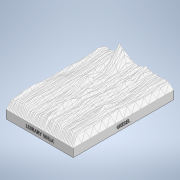
# Autodesk Inventor part: 12_tone_fourier_transform
Saved by Autodesk Inventor 2020 (Build 240168000, 168)
## iProperties
Created: 2019-10-01
Part Number: 12_tone_fourier_transform
Material: Generic
Document SubType Name: Modeling
Designer: Babynado
Density: 1 g/cm^3
Appearance: Default
Author: Babynado
Autodesk Inventor part; units mm, degrees
(part 1 of 4)
ref_plane "YZ Plane" through (0, 0, 0) normal (1, 0, 0) x (0, 1, 0)
ref_plane "XZ Plane" through (0, 0, 0) normal (0, 1, 0) x (-1, 0, 0)
ref_plane "XY Plane" through (0, 0, 0) normal (0, 0, 1) x (1, 0, 0)
sketch "Sketch1" plane through (0, 0, 0) normal (0, 1, 0) x (-1, 0, 0)
  line L0 (-203.2, 304.8) -> (-203.2, 0) projected
  line L1 (0, 304.8) -> (-203.2, 304.8) projected
  line L2 (0, 0) -> (0, 304.8) projected
  line L3 (-203.2, 0) -> (0, 0) projected
extrude "Extrusion1" add sketch "Sketch1" against normal blind 25.4
sketch "Sketch2" plane through (0, 0, 304.8) normal (0, 0, 1) x (1, 0, 0)
  line L0 (0, 0) -> (203.2, 0) projected
  line L1 (0, 0) -> (0, -25.4) projected
  line L2 (203.2, -25.4) -> (0, -25.4) projected
  line L3 (203.2, 0) -> (203.2, -25.4) projected
  line L4 (50.8, -8.636) -> (152.4, -8.636) construction
  line L5 (152.4, -8.636) -> (152.4, -16.764) construction
  line L6 (152.4, -16.764) -> (50.8, -16.764) construction
  line L7 (50.8, -16.764) -> (50.8, -8.636) construction
  line L8 (65.2204, -17.272) -> (59.9222, -17.272)
  line L9 (59.9222, -17.272) -> (59.9222, -8.128)
  line L10 (59.9222, -8.128) -> (61.1374, -8.128)
  line L11 (61.1374, -8.128) -> (61.1374, -16.1901)
  line L12 (61.1374, -16.1901) -> (65.2204, -16.1901)
  line L13 (65.2204, -16.1901) -> (65.2204, -17.272)
  line L14 (69.3626, -17.272) -> (65.8206, -17.272)
  line L15 (65.8206, -17.272) -> (65.8206, -16.3383)
  line L16 (65.8206, -16.3383) -> (66.984, -16.3383)
  line L17 (66.984, -16.3383) -> (66.984, -9.0617)
  line L18 (66.984, -9.0617) -> (65.8206, -9.0617)
  line L19 (65.8206, -9.0617) -> (65.8206, -8.128)
  line L20 (65.8206, -8.128) -> (69.3626, -8.128)
  line L21 (69.3626, -8.128) -> (69.3626, -9.0617)
  line L22 (69.3626, -9.0617) -> (68.1992, -9.0617)
  line L23 (68.1992, -9.0617) -> (68.1992, -16.3383)
  line L24 (68.1992, -16.3383) -> (69.3626, -16.3383)
  line L25 (69.3626, -16.3383) -> (69.3626, -17.272)
  spline S0 degree 2 poles (77.069, -14.4636) (77.069, -15.1453) (76.5503, -16.1901) (76.1205, -16.531) knots 0 0 0 1 2 2 2
  spline S1 degree 2 poles (76.1205, -16.531) (75.6018, -16.9311) (74.4236, -17.272) (73.49, -17.272) knots 0 0 0 1 2 2 2
  line L26 (73.49, -17.272) -> (70.8668, -17.272)
  line L27 (70.8668, -17.272) -> (70.8668, -8.128)
  line L28 (70.8668, -8.128) -> (73.2899, -8.128)
  spline S2 degree 2 poles (73.2899, -8.128) (74.268, -8.128) (75.2462, -8.254) (75.6908, -8.4985) knots 0 0 0 1 2 2 2
  spline S3 degree 2 poles (75.6908, -8.4985) (76.1872, -8.7579) (76.6392, -9.61) (76.6392, -10.188) knots 0 0 0 1 2 2 2
  spline S4 degree 2 poles (76.6392, -10.188) (76.6392, -10.8327) (75.9575, -11.8553) (75.3573, -12.1442) knots 0 0 0 1 2 2 2
  line L29 (75.3573, -12.1442) -> (75.3573, -12.1887)
  spline S5 degree 2 poles (75.3573, -12.1887) (76.1724, -12.411) (77.069, -13.5892) (77.069, -14.4636) knots 0 0 0 1 2 2 2
  spline S6 degree 2 poles (75.8019, -14.5155) (75.8019, -13.9968) (75.5055, -13.3299) (75.0609, -13.0927) knots 0 0 0 1 2 2 2
  spline S7 degree 2 poles (75.0609, -13.0927) (74.7719, -12.9445) (74.0902, -12.8556) (73.4603, -12.8556) knots 0 0 0 1 2 2 2
  line L30 (73.4603, -12.8556) -> (72.0821, -12.8556)
  line L31 (72.0821, -12.8556) -> (72.0821, -16.2346)
  line L32 (72.0821, -16.2346) -> (73.0676, -16.2346)
  spline S8 degree 2 poles (73.0676, -16.2346) (73.8679, -16.2346) (74.7867, -16.0864) (75.1424, -15.8493) knots 0 0 0 1 2 2 2
  spline S9 degree 2 poles (75.1424, -15.8493) (75.4833, -15.6047) (75.8019, -14.9971) (75.8019, -14.5155) knots 0 0 0 1 2 2 2
  spline S10 degree 2 poles (75.3721, -10.3584) (75.3721, -10.0324) (75.1498, -9.5433) (74.9053, -9.4025) knots 0 0 0 1 2 2 2
  spline S11 degree 2 poles (74.9053, -9.4025) (74.6089, -9.2395) (73.8901, -9.1654) (73.2454, -9.1654) knots 0 0 0 1 2 2 2
  line L33 (73.2454, -9.1654) -> (72.0821, -9.1654)
  line L34 (72.0821, -9.1654) -> (72.0821, -11.8404)
  line L35 (72.0821, -11.8404) -> (73.4603, -11.8404)
  spline S12 degree 2 poles (73.4603, -11.8404) (74.0309, -11.8404) (74.5718, -11.7219) (74.8608, -11.5366) knots 0 0 0 1 2 2 2
  spline S13 degree 2 poles (74.8608, -11.5366) (75.1424, -11.3588) (75.3721, -10.7882) (75.3721, -10.3584) knots 0 0 0 1 2 2 2
  line L36 (85.3535, -17.272) -> (83.7751, -17.272)
  line L37 (83.7751, -17.272) -> (80.8852, -13.6337)
  line L38 (80.8852, -13.6337) -> (79.4921, -13.6337)
  line L39 (79.4921, -13.6337) -> (79.4921, -17.272)
  line L40 (79.4921, -17.272) -> (78.2769, -17.272)
  line L41 (78.2769, -17.272) -> (78.2769, -8.128)
  line L42 (78.2769, -8.128) -> (80.6333, -8.128)
  spline S14 degree 2 poles (80.6333, -8.128) (81.4187, -8.128) (82.4784, -8.2984) (82.96, -8.6097) knots 0 0 0 1 2 2 2
  spline S15 degree 2 poles (82.96, -8.6097) (83.4417, -8.9209) (83.9974, -9.8916) (83.9974, -10.6104) knots 0 0 0 1 2 2 2
  spline S16 degree 2 poles (83.9974, -10.6104) (83.9974, -11.6107) (82.9748, -12.9668) (82.1005, -13.2928) knots 0 0 0 1 2 2 2
  line L43 (82.1005, -13.2928) -> (85.3535, -17.272)
  spline S17 degree 2 poles (82.7303, -10.7067) (82.7303, -10.3066) (82.4487, -9.6915) (82.1523, -9.4914) knots 0 0 0 1 2 2 2
  spline S18 degree 2 poles (82.1523, -9.4914) (81.893, -9.321) (81.2038, -9.1802) (80.7, -9.1802) knots 0 0 0 1 2 2 2
  line L44 (80.7, -9.1802) -> (79.4921, -9.1802)
  line L45 (79.4921, -9.1802) -> (79.4921, -12.6185)
  line L46 (79.4921, -12.6185) -> (80.5592, -12.6185)
  spline S19 degree 2 poles (80.5592, -12.6185) (81.0853, -12.6185) (81.9226, -12.4332) (82.2116, -12.1442) knots 0 0 0 1 2 2 2
  spline S20 degree 2 poles (82.2116, -12.1442) (82.4784, -11.8923) (82.7303, -11.1809) (82.7303, -10.7067) knots 0 0 0 1 2 2 2
  line L47 (85.0941, -17.272) -> (88.1767, -8.128)
  line L48 (88.1767, -8.128) -> (89.6735, -8.128)
  line L49 (89.6735, -8.128) -> (92.7561, -17.272)
  line L50 (92.7561, -17.272) -> (91.4742, -17.272)
  line L51 (91.4742, -17.272) -> (90.6442, -14.7155)
  line L52 (90.6442, -14.7155) -> (87.1541, -14.7155)
  line L53 (87.1541, -14.7155) -> (86.3242, -17.272)
  line L54 (86.3242, -17.272) -> (85.0941, -17.272)
  line L55 (90.3108, -13.6781) -> (88.8955, -9.3729)
  line L56 (88.8955, -9.3729) -> (87.4876, -13.6781)
  line L57 (87.4876, -13.6781) -> (90.3108, -13.6781)
  line L58 (100.6997, -17.272) -> (99.1213, -17.272)
  line L59 (99.1213, -17.272) -> (96.2314, -13.6337)
  line L60 (96.2314, -13.6337) -> (94.8383, -13.6337)
  line L61 (94.8383, -13.6337) -> (94.8383, -17.272)
  line L62 (94.8383, -17.272) -> (93.6231, -17.272)
  line L63 (93.6231, -17.272) -> (93.6231, -8.128)
  line L64 (93.6231, -8.128) -> (95.9795, -8.128)
  spline S21 degree 2 poles (95.9795, -8.128) (96.7649, -8.128) (97.8246, -8.2984) (98.3062, -8.6097) knots 0 0 0 1 2 2 2
  spline S22 degree 2 poles (98.3062, -8.6097) (98.7879, -8.9209) (99.3436, -9.8916) (99.3436, -10.6104) knots 0 0 0 1 2 2 2
  spline S23 degree 2 poles (99.3436, -10.6104) (99.3436, -11.6107) (98.3211, -12.9668) (97.4467, -13.2928) knots 0 0 0 1 2 2 2
  line L65 (97.4467, -13.2928) -> (100.6997, -17.272)
  spline S24 degree 2 poles (98.0765, -10.7067) (98.0765, -10.3066) (97.7949, -9.6915) (97.4985, -9.4914) knots 0 0 0 1 2 2 2
  spline S25 degree 2 poles (97.4985, -9.4914) (97.2392, -9.321) (96.55, -9.1802) (96.0462, -9.1802) knots 0 0 0 1 2 2 2
  line L66 (96.0462, -9.1802) -> (94.8383, -9.1802)
  line L67 (94.8383, -9.1802) -> (94.8383, -12.6185)
  line L68 (94.8383, -12.6185) -> (95.9054, -12.6185)
  spline S26 degree 2 poles (95.9054, -12.6185) (96.4315, -12.6185) (97.2688, -12.4332) (97.5578, -12.1442) knots 0 0 0 1 2 2 2
  spline S27 degree 2 poles (97.5578, -12.1442) (97.8246, -11.8923) (98.0765, -11.1809) (98.0765, -10.7067) knots 0 0 0 1 2 2 2
  line L69 (107.8281, -8.128) -> (104.7382, -13.2261)
  line L70 (104.7382, -13.2261) -> (104.7382, -17.272)
  line L71 (104.7382, -17.272) -> (103.5229, -17.272)
  line L72 (103.5229, -17.272) -> (103.5229, -13.3521)
  line L73 (103.5229, -13.3521) -> (100.4329, -8.128)
  line L74 (100.4329, -8.128) -> (101.7815, -8.128)
  line L75 (101.7815, -8.128) -> (104.1379, -12.1517)
  line L76 (104.1379, -12.1517) -> (106.5388, -8.128)
  line L77 (106.5388, -8.128) -> (107.8281, -8.128)
  line L78 (122.8483, -8.128) -> (120.5512, -17.272)
  line L79 (120.5512, -17.272) -> (119.1877, -17.272)
  line L80 (119.1877, -17.272) -> (117.3278, -9.6841)
  line L81 (117.3278, -9.6841) -> (115.5198, -17.272)
  line L82 (115.5198, -17.272) -> (114.1711, -17.272)
  line L83 (114.1711, -17.272) -> (111.837, -8.128)
  line L84 (111.837, -8.128) -> (113.0893, -8.128)
  line L85 (113.0893, -8.128) -> (114.927, -15.7085)
  line L86 (114.927, -15.7085) -> (116.7498, -8.128)
  line L87 (116.7498, -8.128) -> (117.9873, -8.128)
  line L88 (117.9873, -8.128) -> (119.825, -15.7974)
  line L89 (119.825, -15.7974) -> (121.6553, -8.128)
  line L90 (121.6553, -8.128) -> (122.8483, -8.128)
  line L91 (122.9521, -17.272) -> (126.0346, -8.128)
  line L92 (126.0346, -8.128) -> (127.5315, -8.128)
  line L93 (127.5315, -8.128) -> (130.614, -17.272)
  line L94 (130.614, -17.272) -> (129.3321, -17.272)
  line L95 (129.3321, -17.272) -> (128.5022, -14.7155)
  line L96 (128.5022, -14.7155) -> (125.012, -14.7155)
  line L97 (125.012, -14.7155) -> (124.1821, -17.272)
  line L98 (124.1821, -17.272) -> (122.9521, -17.272)
  line L99 (128.1687, -13.6781) -> (126.7534, -9.3729)
  line L100 (126.7534, -9.3729) -> (125.3455, -13.6781)
  line L101 (125.3455, -13.6781) -> (128.1687, -13.6781)
  line L102 (136.7792, -17.272) -> (131.481, -17.272)
  line L103 (131.481, -17.272) -> (131.481, -8.128)
  line L104 (131.481, -8.128) -> (132.6963, -8.128)
  line L105 (132.6963, -8.128) -> (132.6963, -16.1901)
  line L106 (132.6963, -16.1901) -> (136.7792, -16.1901)
  line L107 (136.7792, -16.1901) -> (136.7792, -17.272)
  line L108 (144.4041, -17.272) -> (142.8258, -17.272)
  line L109 (142.8258, -17.272) -> (139.4839, -13.0186)
  line L110 (139.4839, -13.0186) -> (138.9503, -13.6188)
  line L111 (138.9503, -13.6188) -> (138.9503, -17.272)
  line L112 (138.9503, -17.272) -> (137.7351, -17.272)
  line L113 (137.7351, -17.272) -> (137.7351, -8.128)
  line L114 (137.7351, -8.128) -> (138.9503, -8.128)
  line L115 (138.9503, -8.128) -> (138.9503, -12.3295)
  line L116 (138.9503, -12.3295) -> (142.6998, -8.128)
  line L117 (142.6998, -8.128) -> (144.1818, -8.128)
  line L118 (144.1818, -8.128) -> (140.3953, -12.2109)
  line L119 (140.3953, -12.2109) -> (144.4041, -17.272)
  dimension "d2" = 203.2
  dimension "d3" = 25.4
  dimension "d4" = 101.6
  dimension "d5" = 8.128
  dimension "d6" = 50.8
  dimension "d7" = 8.636
  constraints: 2 other
  measures "d2" distance of L0.start L0.end
  measures "d3" distance of L0.start L1.end
  measures "d4" distance of L4.start L4.end
  measures "d5" distance of L6.end L4.start
  measures "d6" distance between parallel lines of L1 L7
  measures "d7" distance between parallel lines of L2 L6
extrude "Extrusion2" cut sketch "Sketch2" against normal blind 5.08 contours L8 L9 L10 L11 L12 L13 | L14 L15 L16 L17 L18 L19 L20 L21 L22 L23 L24 L25 | S0 S1 L26 L27 L28 S2 S3 S4 L29 S5 | L36 L47 L43 | L43 L47 L48 L49 L50 L51 L52 L53 L54 | L36 L37 L38 L39 L40 L41 L42 S14 S15 S16 L43 L47 | L58 L59 L60 L61 L62 L63 L64 S21 S22 S23 L65 | L69 L70 L71 L72 L73 L74 L75 L76 L77 | L78 L79 L80 L81 L82 L83 L84 L85 L86 L87 L88 L89 L90 | L91 L92 L93 L94 L95 L96 L97 L98 | L102 L103 L104 L105 L106 L107 | L108 L109 L110 L111 L112 L113 L114 L115 L116 L117 L118 L119
sketch "Sketch3" plane through (203.2, 0, 304.8) normal (1, 0, 0) x (0, 0, -1)
  line L0 (0, 0) -> (304.8, 0) projected
  line L1 (0, 0) -> (0, -25.4) projected
  line L2 (304.8, -25.4) -> (0, -25.4) projected
  line L3 (304.8, 0) -> (304.8, -25.4) projected
  line L4 (120.65, -8.636) -> (184.15, -8.636) construction
  line L5 (184.15, -8.636) -> (184.15, -16.764) construction
  line L6 (184.15, -16.764) -> (120.65, -16.764) construction
  line L7 (120.65, -16.764) -> (120.65, -8.636) construction
  spline S0 degree 2 poles (136.9315, -17.4424) (135.9608, -17.4424) (134.3528, -16.8496) (133.7748, -16.2494) knots 0 0 0 1 2 2 2
  spline S1 degree 2 poles (133.7748, -16.2494) (133.1969, -15.6418) (132.5818, -13.8486) (132.5818, -12.6852) knots 0 0 0 1 2 2 2
  spline S2 degree 2 poles (132.5818, -12.6852) (132.5818, -11.5811) (133.2043, -9.8323) (133.7823, -9.2099) knots 0 0 0 1 2 2 2
  spline S3 degree 2 poles (133.7823, -9.2099) (134.338, -8.6097) (135.9682, -7.9576) (136.9389, -7.9576) knots 0 0 0 1 2 2 2
  spline S4 degree 2 poles (136.9389, -7.9576) (137.4058, -7.9576) (138.2505, -8.0909) (138.6358, -8.2095) knots 0 0 0 1 2 2 2
  spline S5 degree 2 poles (138.6358, -8.2095) (138.9471, -8.2984) (139.7029, -8.6245) (139.9326, -8.743) knots 0 0 0 1 2 2 2
  line L8 (139.9326, -8.743) -> (139.9326, -10.2102)
  line L9 (139.9326, -10.2102) -> (139.8289, -10.2102)
  spline S6 degree 2 poles (139.8289, -10.2102) (139.5991, -10.0102) (139.1175, -9.6471) (138.6729, -9.4396) knots 0 0 0 1 2 2 2
  spline S7 degree 2 poles (138.6729, -9.4396) (138.3024, -9.2543) (137.3465, -9.0098) (136.7981, -9.0098) knots 0 0 0 1 2 2 2
  spline S8 degree 2 poles (136.7981, -9.0098) (135.4792, -9.0098) (133.8489, -10.9957) (133.8489, -12.6481) knots 0 0 0 1 2 2 2
  spline S9 degree 2 poles (133.8489, -12.6481) (133.8489, -13.567) (134.2787, -14.9452) (134.6863, -15.4195) knots 0 0 0 1 2 2 2
  spline S10 degree 2 poles (134.6863, -15.4195) (135.079, -15.8937) (136.1905, -16.3902) (136.8871, -16.3902) knots 0 0 0 1 2 2 2
  spline S11 degree 2 poles (136.8871, -16.3902) (137.3984, -16.3902) (138.4209, -16.242) (138.7692, -16.0938) knots 0 0 0 1 2 2 2
  line L10 (138.7692, -16.0938) -> (138.7692, -13.73)
  line L11 (138.7692, -13.73) -> (136.6499, -13.73)
  line L12 (136.6499, -13.73) -> (136.6499, -12.6629)
  line L13 (136.6499, -12.6629) -> (139.9696, -12.6629)
  line L14 (139.9696, -12.6629) -> (139.9696, -16.657)
  spline S12 degree 2 poles (139.9696, -16.657) (139.7399, -16.7607) (138.9545, -17.0793) (138.621, -17.1757) knots 0 0 0 1 2 2 2
  spline S13 degree 2 poles (138.621, -17.1757) (138.169, -17.3091) (137.4428, -17.4424) (136.9315, -17.4424) knots 0 0 0 1 2 2 2
  line L15 (141.4961, -17.2646) -> (141.4961, -8.1206)
  line L16 (141.4961, -8.1206) -> (147.2167, -8.1206)
  line L17 (147.2167, -8.1206) -> (147.2167, -9.2025)
  line L18 (147.2167, -9.2025) -> (142.7114, -9.2025)
  line L19 (142.7114, -9.2025) -> (142.7114, -11.7071)
  line L20 (142.7114, -11.7071) -> (146.9129, -11.7071)
  line L21 (146.9129, -11.7071) -> (146.9129, -12.7889)
  line L22 (146.9129, -12.7889) -> (142.7114, -12.7889)
  line L23 (142.7114, -12.7889) -> (142.7114, -16.1827)
  line L24 (142.7114, -16.1827) -> (147.2167, -16.1827)
  line L25 (147.2167, -16.1827) -> (147.2167, -17.2646)
  line L26 (147.2167, -17.2646) -> (141.4961, -17.2646)
  line L27 (151.7368, -17.2646) -> (148.1948, -17.2646)
  line L28 (148.1948, -17.2646) -> (148.1948, -16.3309)
  line L29 (148.1948, -16.3309) -> (149.3582, -16.3309)
  line L30 (149.3582, -16.3309) -> (149.3582, -9.0543)
  line L31 (149.3582, -9.0543) -> (148.1948, -9.0543)
  line L32 (148.1948, -9.0543) -> (148.1948, -8.1206)
  line L33 (148.1948, -8.1206) -> (151.7368, -8.1206)
  line L34 (151.7368, -8.1206) -> (151.7368, -9.0543)
  line L35 (151.7368, -9.0543) -> (150.5734, -9.0543)
  line L36 (150.5734, -9.0543) -> (150.5734, -16.3309)
  line L37 (150.5734, -16.3309) -> (151.7368, -16.3309)
  line L38 (151.7368, -16.3309) -> (151.7368, -17.2646)
  spline S14 degree 2 poles (155.7901, -17.4276) (154.7971, -17.4276) (153.4041, -17.0126) (152.789, -16.7162) knots 0 0 0 1 2 2 2
  line L39 (152.789, -16.7162) -> (152.789, -15.1898)
  line L40 (152.789, -15.1898) -> (152.8779, -15.1898)
  spline S15 degree 2 poles (152.8779, -15.1898) (153.4782, -15.7529) (154.9972, -16.3754) (155.7012, -16.3754) knots 0 0 0 1 2 2 2
  spline S16 degree 2 poles (155.7012, -16.3754) (156.7089, -16.3754) (157.7389, -15.538) (157.7389, -14.8489) knots 0 0 0 1 2 2 2
  spline S17 degree 2 poles (157.7389, -14.8489) (157.7389, -14.3006) (157.198, -13.6188) (156.6126, -13.4484) knots 0 0 0 1 2 2 2
  spline S18 degree 2 poles (156.6126, -13.4484) (156.1902, -13.3299) (155.4863, -13.1668) (154.9602, -13.0335) knots 0 0 0 1 2 2 2
  spline S19 degree 2 poles (154.9602, -13.0335) (154.4859, -12.9075) (153.7375, -12.5296) (153.4485, -12.2258) knots 0 0 0 1 2 2 2
  spline S20 degree 2 poles (153.4485, -12.2258) (153.1669, -11.9219) (152.8557, -11.1068) (152.8557, -10.5733) knots 0 0 0 1 2 2 2
  spline S21 degree 2 poles (152.8557, -10.5733) (152.8557, -9.4618) (154.5897, -7.9576) (155.9309, -7.9576) knots 0 0 0 1 2 2 2
  spline S22 degree 2 poles (155.9309, -7.9576) (156.7015, -7.9576) (158.065, -8.2614) (158.6504, -8.5504) knots 0 0 0 1 2 2 2
  line L41 (158.6504, -8.5504) -> (158.6504, -10.0027)
  line L42 (158.6504, -10.0027) -> (158.5615, -10.0027)
  spline S23 degree 2 poles (158.5615, -10.0027) (158.1243, -9.6026) (156.7608, -9.0098) (156.0124, -9.0098) knots 0 0 0 1 2 2 2
  spline S24 degree 2 poles (156.0124, -9.0098) (155.1677, -9.0098) (154.1228, -9.8027) (154.1228, -10.4473) knots 0 0 0 1 2 2 2
  spline S25 degree 2 poles (154.1228, -10.4473) (154.1228, -11.0253) (154.7379, -11.7145) (155.3159, -11.8701) knots 0 0 0 1 2 2 2
  spline S26 degree 2 poles (155.3159, -11.8701) (155.7012, -11.9738) (156.8201, -12.2406) (157.1906, -12.3517) knots 0 0 0 1 2 2 2
  spline S27 degree 2 poles (157.1906, -12.3517) (158.1317, -12.6407) (159.0061, -13.8041) (159.0061, -14.6563) knots 0 0 0 1 2 2 2
  spline S28 degree 2 poles (159.0061, -14.6563) (159.0061, -15.1972) (158.5689, -16.2346) (158.1761, -16.5977) knots 0 0 0 1 2 2 2
  spline S29 degree 2 poles (158.1761, -16.5977) (157.7389, -16.9978) (156.6274, -17.4276) (155.7901, -17.4276) knots 0 0 0 1 2 2 2
  line L43 (160.2435, -17.2646) -> (160.2435, -8.1206)
  line L44 (160.2435, -8.1206) -> (165.9641, -8.1206)
  line L45 (165.9641, -8.1206) -> (165.9641, -9.2025)
  line L46 (165.9641, -9.2025) -> (161.4588, -9.2025)
  line L47 (161.4588, -9.2025) -> (161.4588, -11.7071)
  line L48 (161.4588, -11.7071) -> (165.6603, -11.7071)
  line L49 (165.6603, -11.7071) -> (165.6603, -12.7889)
  line L50 (165.6603, -12.7889) -> (161.4588, -12.7889)
  line L51 (161.4588, -12.7889) -> (161.4588, -16.1827)
  line L52 (161.4588, -16.1827) -> (165.9641, -16.1827)
  line L53 (165.9641, -16.1827) -> (165.9641, -17.2646)
  line L54 (165.9641, -17.2646) -> (160.2435, -17.2646)
  line L55 (172.5961, -17.2646) -> (167.2979, -17.2646)
  line L56 (167.2979, -17.2646) -> (167.2979, -8.1206)
  line L57 (167.2979, -8.1206) -> (168.5131, -8.1206)
  line L58 (168.5131, -8.1206) -> (168.5131, -16.1827)
  line L59 (168.5131, -16.1827) -> (172.5961, -16.1827)
  line L60 (172.5961, -16.1827) -> (172.5961, -17.2646)
  dimension "d10" = 304.8
  dimension "d11" = 25.4
  dimension "d12" = 63.5
  dimension "d13" = 8.128
  dimension "d14" = 120.65
  dimension "d15" = 8.636
  constraints: 2 other
  measures "d10" distance of L0.start L0.end
  measures "d11" distance of L0.start L1.end
  measures "d12" distance of L4.start L4.end
  measures "d13" distance of L6.end L4.start
  measures "d14" distance between parallel lines of L1 L7
  measures "d15" distance between parallel lines of L2 L6
extrude "Extrusion3" cut sketch "Sketch3" against normal blind 5.08 contours S0 S1 S2 S3 S4 S5 L8 L9 S6 S7 S8 S9 S10 S11 L10 L11 L12 L13 L14 S12 S13 | L15 L16 L17 L18 L19 L20 L21 L22 L23 L24 L25 L26 | L27 L28 L29 L30 L31 L32 L33 L34 L35 L36 L37 L38 | S14 L39 L40 S15 S16 S17 S18 S19 S20 S21 S22 L41 L42 S23 S24 S25 S26 S27 S28 S29 | L43 L44 L45 L46 L47 L48 L49 L50 L51 L52 L53 L54 | L55 L56 L57 L58 L59 L60
sketch "Sketch4" plane through (203.2, 0, 0) normal (0, 0, -1) x (-1, 0, 0)
  line L0 (10.16, -7.62) -> (193.04, -7.62) construction
  line L1 (193.04, -7.62) -> (193.04, -17.78) construction
  line L2 (193.04, -17.78) -> (10.16, -17.78) construction
  line L3 (10.16, -17.78) -> (10.16, -7.62) construction
  line L4 (0, 0) -> (203.2, 0) projected
  line L5 (0, 0) -> (0, -25.4) projected
  line L6 (203.2, -25.4) -> (0, -25.4) projected
  line L7 (203.2, 0) -> (203.2, -25.4) projected
  line L8 (17.4811, -17.272) -> (13.0203, -17.272)
  line L9 (13.0203, -17.272) -> (13.0203, -16.3383)
  line L10 (13.0203, -16.3383) -> (14.6801, -16.3383)
  line L11 (14.6801, -16.3383) -> (14.6801, -10.2102)
  line L12 (14.6801, -10.2102) -> (13.0203, -10.2102)
  line L13 (13.0203, -10.2102) -> (13.0203, -9.3729)
  spline S0 degree 2 poles (13.0203, -9.3729) (13.9614, -9.3729) (14.8506, -8.8394) (14.9098, -8.0984) knots 0 0 0 1 2 2 2
  line L14 (14.9098, -8.0984) -> (15.8583, -8.0984)
  line L15 (15.8583, -8.0984) -> (15.8583, -16.3383)
  line L16 (15.8583, -16.3383) -> (17.4811, -16.3383)
  line L17 (17.4811, -16.3383) -> (17.4811, -17.272)
  line L18 (24.8023, -17.272) -> (19.1632, -17.272)
  line L19 (19.1632, -17.272) -> (19.1632, -15.9752)
  spline S1 degree 2 poles (19.1632, -15.9752) (19.7708, -15.4047) (20.8527, -14.345) (21.3714, -13.7745) knots 0 0 0 1 2 2 2
  spline S2 degree 2 poles (21.3714, -13.7745) (22.4162, -12.6259) (23.1795, -11.2476) (23.1795, -10.514) knots 0 0 0 1 2 2 2
  spline S3 degree 2 poles (23.1795, -10.514) (23.1795, -10.1287) (22.9423, -9.5507) (22.7274, -9.3655) knots 0 0 0 1 2 2 2
  spline S4 degree 2 poles (22.7274, -9.3655) (22.5125, -9.1802) (21.9494, -8.995) (21.6085, -8.995) knots 0 0 0 1 2 2 2
  spline S5 degree 2 poles (21.6085, -8.995) (21.2825, -8.995) (20.6156, -9.158) (20.3118, -9.284) knots 0 0 0 1 2 2 2
  spline S6 degree 2 poles (20.3118, -9.284) (20.0524, -9.3877) (19.5708, -9.6841) (19.4226, -9.7879) knots 0 0 0 1 2 2 2
  line L20 (19.4226, -9.7879) -> (19.3559, -9.7879)
  line L21 (19.3559, -9.7879) -> (19.3559, -8.4837)
  spline S7 degree 2 poles (19.3559, -8.4837) (19.7338, -8.2984) (21.0898, -7.9353) (21.6974, -7.9353) knots 0 0 0 1 2 2 2
  spline S8 degree 2 poles (21.6974, -7.9353) (22.9794, -7.9353) (24.4243, -9.2914) (24.4243, -10.4473) knots 0 0 0 1 2 2 2
  spline S9 degree 2 poles (24.4243, -10.4473) (24.4243, -10.9883) (24.1724, -11.8923) (23.9501, -12.2776) knots 0 0 0 1 2 2 2
  spline S10 degree 2 poles (23.9501, -12.2776) (23.7278, -12.6778) (23.0831, -13.4632) (22.7274, -13.8411) knots 0 0 0 1 2 2 2
  spline S11 degree 2 poles (22.7274, -13.8411) (22.1495, -14.471) (20.7341, -15.8196) (20.3118, -16.2124) knots 0 0 0 1 2 2 2
  line L22 (20.3118, -16.2124) -> (24.8023, -16.2124)
  line L23 (24.8023, -16.2124) -> (24.8023, -17.272)
  line L24 (29.3743, -13.8263) -> (25.9138, -13.8263)
  line L25 (25.9138, -13.8263) -> (25.9138, -12.7148)
  line L26 (25.9138, -12.7148) -> (29.3743, -12.7148)
  line L27 (29.3743, -12.7148) -> (29.3743, -13.8263)
  line L28 (32.9829, -17.272) -> (32.9829, -9.2099)
  line L29 (32.9829, -9.2099) -> (29.9152, -9.2099)
  line L30 (29.9152, -9.2099) -> (29.9152, -8.128)
  line L31 (29.9152, -8.128) -> (37.266, -8.128)
  line L32 (37.266, -8.128) -> (37.266, -9.2099)
  line L33 (37.266, -9.2099) -> (34.1982, -9.2099)
  line L34 (34.1982, -9.2099) -> (34.1982, -17.272)
  line L35 (34.1982, -17.272) -> (32.9829, -17.272)
  spline S12 degree 2 poles (44.6612, -9.1728) (45.1799, -9.7804) (45.7579, -11.5589) (45.7579, -12.7) knots 0 0 0 1 2 2 2
  spline S13 degree 2 poles (45.7579, -12.7) (45.7579, -13.8115) (45.1947, -15.6121) (44.6612, -16.2198) knots 0 0 0 1 2 2 2
  spline S14 degree 2 poles (44.6612, -16.2198) (44.098, -16.857) (42.6086, -17.4647) (41.712, -17.4647) knots 0 0 0 1 2 2 2
  spline S15 degree 2 poles (41.712, -17.4647) (40.7857, -17.4647) (39.3037, -16.8348) (38.7628, -16.2198) knots 0 0 0 1 2 2 2
  spline S16 degree 2 poles (38.7628, -16.2198) (38.2367, -15.6121) (37.6735, -13.8263) (37.6735, -12.7) knots 0 0 0 1 2 2 2
  spline S17 degree 2 poles (37.6735, -12.7) (37.6735, -11.5514) (38.2441, -9.8027) (38.7702, -9.1728) knots 0 0 0 1 2 2 2
  spline S18 degree 2 poles (38.7702, -9.1728) (39.3037, -8.5652) (40.7931, -7.9353) (41.712, -7.9353) knots 0 0 0 1 2 2 2
  spline S19 degree 2 poles (41.712, -7.9353) (42.6457, -7.9353) (44.1425, -8.5874) (44.6612, -9.1728) knots 0 0 0 1 2 2 2
  spline S20 degree 2 poles (44.4908, -12.7) (44.4908, -11.796) (44.098, -10.3955) (43.7423, -9.9361) knots 0 0 0 1 2 2 2
  spline S21 degree 2 poles (43.7423, -9.9361) (43.3792, -9.4618) (42.3567, -8.9876) (41.7194, -8.9876) knots 0 0 0 1 2 2 2
  spline S22 degree 2 poles (41.7194, -8.9876) (41.0599, -8.9876) (40.067, -9.447) (39.689, -9.9361) knots 0 0 0 1 2 2 2
  spline S23 degree 2 poles (39.689, -9.9361) (39.3259, -10.4029) (38.9406, -11.8108) (38.9406, -12.7) knots 0 0 0 1 2 2 2
  spline S24 degree 2 poles (38.9406, -12.7) (38.9406, -14.5006) (40.4523, -16.4124) (41.7194, -16.4124) knots 0 0 0 1 2 2 2
  spline S25 degree 2 poles (41.7194, -16.4124) (42.9865, -16.4124) (44.4908, -14.5006) (44.4908, -12.7) knots 0 0 0 1 2 2 2
  line L36 (53.6348, -17.272) -> (52.2713, -17.272)
  line L37 (52.2713, -17.272) -> (48.2254, -9.3877)
  line L38 (48.2254, -9.3877) -> (48.2254, -17.272)
  line L39 (48.2254, -17.272) -> (47.0917, -17.272)
  line L40 (47.0917, -17.272) -> (47.0917, -8.128)
  line L41 (47.0917, -8.128) -> (48.8182, -8.128)
  line L42 (48.8182, -8.128) -> (52.501, -15.3676)
  line L43 (52.501, -15.3676) -> (52.501, -8.128)
  line L44 (52.501, -8.128) -> (53.6348, -8.128)
  line L45 (53.6348, -8.128) -> (53.6348, -17.272)
  line L46 (55.4873, -17.272) -> (55.4873, -8.128)
  line L47 (55.4873, -8.128) -> (61.2078, -8.128)
  line L48 (61.2078, -8.128) -> (61.2078, -9.2099)
  line L49 (61.2078, -9.2099) -> (56.7025, -9.2099)
  line L50 (56.7025, -9.2099) -> (56.7025, -11.7145)
  line L51 (56.7025, -11.7145) -> (60.904, -11.7145)
  line L52 (60.904, -11.7145) -> (60.904, -12.7963)
  line L53 (60.904, -12.7963) -> (56.7025, -12.7963)
  line L54 (56.7025, -12.7963) -> (56.7025, -16.1901)
  line L55 (56.7025, -16.1901) -> (61.2078, -16.1901)
  line L56 (61.2078, -16.1901) -> (61.2078, -17.272)
  line L57 (61.2078, -17.272) -> (55.4873, -17.272)
  line L58 (71.9376, -9.2099) -> (67.6842, -9.2099)
  line L59 (67.6842, -9.2099) -> (67.6842, -11.7886)
  line L60 (67.6842, -11.7886) -> (71.7597, -11.7886)
  line L61 (71.7597, -11.7886) -> (71.7597, -12.8704)
  line L62 (71.7597, -12.8704) -> (67.6842, -12.8704)
  line L63 (67.6842, -12.8704) -> (67.6842, -17.272)
  line L64 (67.6842, -17.272) -> (66.469, -17.272)
  line L65 (66.469, -17.272) -> (66.469, -8.128)
  line L66 (66.469, -8.128) -> (71.9376, -8.128)
  line L67 (71.9376, -8.128) -> (71.9376, -9.2099)
  spline S26 degree 2 poles (79.4958, -9.1728) (80.0145, -9.7804) (80.5925, -11.5589) (80.5925, -12.7) knots 0 0 0 1 2 2 2
  spline S27 degree 2 poles (80.5925, -12.7) (80.5925, -13.8115) (80.0293, -15.6121) (79.4958, -16.2198) knots 0 0 0 1 2 2 2
  spline S28 degree 2 poles (79.4958, -16.2198) (78.9327, -16.857) (77.4432, -17.4647) (76.5466, -17.4647) knots 0 0 0 1 2 2 2
  spline S29 degree 2 poles (76.5466, -17.4647) (75.6204, -17.4647) (74.1384, -16.8348) (73.5974, -16.2198) knots 0 0 0 1 2 2 2
  spline S30 degree 2 poles (73.5974, -16.2198) (73.0713, -15.6121) (72.5081, -13.8263) (72.5081, -12.7) knots 0 0 0 1 2 2 2
  spline S31 degree 2 poles (72.5081, -12.7) (72.5081, -11.5514) (73.0787, -9.8027) (73.6048, -9.1728) knots 0 0 0 1 2 2 2
  spline S32 degree 2 poles (73.6048, -9.1728) (74.1384, -8.5652) (75.6278, -7.9353) (76.5466, -7.9353) knots 0 0 0 1 2 2 2
  spline S33 degree 2 poles (76.5466, -7.9353) (77.4803, -7.9353) (78.9771, -8.5874) (79.4958, -9.1728) knots 0 0 0 1 2 2 2
  spline S34 degree 2 poles (79.3254, -12.7) (79.3254, -11.796) (78.9327, -10.3955) (78.577, -9.9361) knots 0 0 0 1 2 2 2
  spline S35 degree 2 poles (78.577, -9.9361) (78.2139, -9.4618) (77.1913, -8.9876) (76.554, -8.9876) knots 0 0 0 1 2 2 2
  spline S36 degree 2 poles (76.554, -8.9876) (75.8945, -8.9876) (74.9016, -9.447) (74.5237, -9.9361) knots 0 0 0 1 2 2 2
  spline S37 degree 2 poles (74.5237, -9.9361) (74.1606, -10.4029) (73.7753, -11.8108) (73.7753, -12.7) knots 0 0 0 1 2 2 2
  spline S38 degree 2 poles (73.7753, -12.7) (73.7753, -14.5006) (75.2869, -16.4124) (76.554, -16.4124) knots 0 0 0 1 2 2 2
  spline S39 degree 2 poles (76.554, -16.4124) (77.8212, -16.4124) (79.3254, -14.5006) (79.3254, -12.7) knots 0 0 0 1 2 2 2
  spline S40 degree 2 poles (85.12, -17.4647) (84.3124, -17.4647) (83.1119, -17.0423) (82.6896, -16.6199) knots 0 0 0 1 2 2 2
  spline S41 degree 2 poles (82.6896, -16.6199) (82.2079, -16.1457) (81.8152, -14.8119) (81.8152, -13.8337) knots 0 0 0 1 2 2 2
  line L68 (81.8152, -13.8337) -> (81.8152, -8.128)
  line L69 (81.8152, -8.128) -> (83.0304, -8.128)
  line L70 (83.0304, -8.128) -> (83.0304, -13.8337)
  spline S42 degree 2 poles (83.0304, -13.8337) (83.0304, -14.471) (83.1934, -15.3306) (83.4231, -15.6788) knots 0 0 0 1 2 2 2
  spline S43 degree 2 poles (83.4231, -15.6788) (83.6677, -16.0493) (84.5124, -16.4273) (85.12, -16.4273) knots 0 0 0 1 2 2 2
  spline S44 degree 2 poles (85.12, -16.4273) (85.6906, -16.4273) (86.5798, -16.0493) (86.8244, -15.6788) knots 0 0 0 1 2 2 2
  spline S45 degree 2 poles (86.8244, -15.6788) (87.0541, -15.3306) (87.2171, -14.4784) (87.2171, -13.8634) knots 0 0 0 1 2 2 2
  line L71 (87.2171, -13.8634) -> (87.2171, -8.128)
  line L72 (87.2171, -8.128) -> (88.4323, -8.128)
  line L73 (88.4323, -8.128) -> (88.4323, -13.8337)
  spline S46 degree 2 poles (88.4323, -13.8337) (88.4323, -14.7896) (88.047, -16.1531) (87.558, -16.6199) knots 0 0 0 1 2 2 2
  spline S47 degree 2 poles (87.558, -16.6199) (87.1208, -17.0497) (85.9648, -17.4647) (85.12, -17.4647) knots 0 0 0 1 2 2 2
  line L74 (97.2503, -17.272) -> (95.672, -17.272)
  line L75 (95.672, -17.272) -> (92.782, -13.6337)
  line L76 (92.782, -13.6337) -> (91.3889, -13.6337)
  line L77 (91.3889, -13.6337) -> (91.3889, -17.272)
  line L78 (91.3889, -17.272) -> (90.1737, -17.272)
  line L79 (90.1737, -17.272) -> (90.1737, -8.128)
  line L80 (90.1737, -8.128) -> (92.5301, -8.128)
  spline S48 degree 2 poles (92.5301, -8.128) (93.3156, -8.128) (94.3752, -8.2984) (94.8569, -8.6097) knots 0 0 0 1 2 2 2
  spline S49 degree 2 poles (94.8569, -8.6097) (95.3385, -8.9209) (95.8943, -9.8916) (95.8943, -10.6104) knots 0 0 0 1 2 2 2
  spline S50 degree 2 poles (95.8943, -10.6104) (95.8943, -11.6107) (94.8717, -12.9668) (93.9973, -13.2928) knots 0 0 0 1 2 2 2
  line L81 (93.9973, -13.2928) -> (97.2503, -17.272)
  spline S51 degree 2 poles (94.6271, -10.7067) (94.6271, -10.3066) (94.3456, -9.6915) (94.0492, -9.4914) knots 0 0 0 1 2 2 2
  spline S52 degree 2 poles (94.0492, -9.4914) (93.7898, -9.321) (93.1007, -9.1802) (92.5968, -9.1802) knots 0 0 0 1 2 2 2
  line L82 (92.5968, -9.1802) -> (91.3889, -9.1802)
  line L83 (91.3889, -9.1802) -> (91.3889, -12.6185)
  line L84 (91.3889, -12.6185) -> (92.456, -12.6185)
  spline S53 degree 2 poles (92.456, -12.6185) (92.9821, -12.6185) (93.8194, -12.4332) (94.1084, -12.1442) knots 0 0 0 1 2 2 2
  spline S54 degree 2 poles (94.1084, -12.1442) (94.3752, -11.8923) (94.6271, -11.1809) (94.6271, -10.7067) knots 0 0 0 1 2 2 2
  line L85 (101.1628, -17.272) -> (97.6208, -17.272)
  line L86 (97.6208, -17.272) -> (97.6208, -16.3383)
  line L87 (97.6208, -16.3383) -> (98.7842, -16.3383)
  line L88 (98.7842, -16.3383) -> (98.7842, -9.0617)
  line L89 (98.7842, -9.0617) -> (97.6208, -9.0617)
  line L90 (97.6208, -9.0617) -> (97.6208, -8.128)
  line L91 (97.6208, -8.128) -> (101.1628, -8.128)
  line L92 (101.1628, -8.128) -> (101.1628, -9.0617)
  line L93 (101.1628, -9.0617) -> (99.9994, -9.0617)
  line L94 (99.9994, -9.0617) -> (99.9994, -16.3383)
  line L95 (99.9994, -16.3383) -> (101.1628, -16.3383)
  line L96 (101.1628, -16.3383) -> (101.1628, -17.272)
  line L97 (102.667, -17.272) -> (102.667, -8.128)
  line L98 (102.667, -8.128) -> (108.3876, -8.128)
  line L99 (108.3876, -8.128) -> (108.3876, -9.2099)
  line L100 (108.3876, -9.2099) -> (103.8823, -9.2099)
  line L101 (103.8823, -9.2099) -> (103.8823, -11.7145)
  line L102 (103.8823, -11.7145) -> (108.0838, -11.7145)
  line L103 (108.0838, -11.7145) -> (108.0838, -12.7963)
  line L104 (108.0838, -12.7963) -> (103.8823, -12.7963)
  line L105 (103.8823, -12.7963) -> (103.8823, -16.1901)
  line L106 (103.8823, -16.1901) -> (108.3876, -16.1901)
  line L107 (108.3876, -16.1901) -> (108.3876, -17.272)
  line L108 (108.3876, -17.272) -> (102.667, -17.272)
  line L109 (116.798, -17.272) -> (115.2197, -17.272)
  line L110 (115.2197, -17.272) -> (112.3297, -13.6337)
  line L111 (112.3297, -13.6337) -> (110.9367, -13.6337)
  line L112 (110.9367, -13.6337) -> (110.9367, -17.272)
  line L113 (110.9367, -17.272) -> (109.7214, -17.272)
  line L114 (109.7214, -17.272) -> (109.7214, -8.128)
  line L115 (109.7214, -8.128) -> (112.0778, -8.128)
  spline S55 degree 2 poles (112.0778, -8.128) (112.8633, -8.128) (113.9229, -8.2984) (114.4046, -8.6097) knots 0 0 0 1 2 2 2
  spline S56 degree 2 poles (114.4046, -8.6097) (114.8862, -8.9209) (115.442, -9.8916) (115.442, -10.6104) knots 0 0 0 1 2 2 2
  spline S57 degree 2 poles (115.442, -10.6104) (115.442, -11.6107) (114.4194, -12.9668) (113.545, -13.2928) knots 0 0 0 1 2 2 2
  line L116 (113.545, -13.2928) -> (116.798, -17.272)
  spline S58 degree 2 poles (114.1748, -10.7067) (114.1748, -10.3066) (113.8933, -9.6915) (113.5969, -9.4914) knots 0 0 0 1 2 2 2
  spline S59 degree 2 poles (113.5969, -9.4914) (113.3375, -9.321) (112.6484, -9.1802) (112.1445, -9.1802) knots 0 0 0 1 2 2 2
  line L117 (112.1445, -9.1802) -> (110.9367, -9.1802)
  line L118 (110.9367, -9.1802) -> (110.9367, -12.6185)
  line L119 (110.9367, -12.6185) -> (112.0037, -12.6185)
  spline S60 degree 2 poles (112.0037, -12.6185) (112.5298, -12.6185) (113.3672, -12.4332) (113.6561, -12.1442) knots 0 0 0 1 2 2 2
  spline S61 degree 2 poles (113.6561, -12.1442) (113.9229, -11.8923) (114.1748, -11.1809) (114.1748, -10.7067) knots 0 0 0 1 2 2 2
  line L120 (123.5856, -17.272) -> (123.5856, -9.2099)
  line L121 (123.5856, -9.2099) -> (120.5179, -9.2099)
  line L122 (120.5179, -9.2099) -> (120.5179, -8.128)
  line L123 (120.5179, -8.128) -> (127.8686, -8.128)
  line L124 (127.8686, -8.128) -> (127.8686, -9.2099)
  line L125 (127.8686, -9.2099) -> (124.8009, -9.2099)
  line L126 (124.8009, -9.2099) -> (124.8009, -17.272)
  line L127 (124.8009, -17.272) -> (123.5856, -17.272)
  line L128 (135.8715, -17.272) -> (134.2931, -17.272)
  line L129 (134.2931, -17.272) -> (131.4032, -13.6337)
  line L130 (131.4032, -13.6337) -> (130.0101, -13.6337)
  line L131 (130.0101, -13.6337) -> (130.0101, -17.272)
  line L132 (130.0101, -17.272) -> (128.7949, -17.272)
  line L133 (128.7949, -17.272) -> (128.7949, -8.128)
  line L134 (128.7949, -8.128) -> (131.1513, -8.128)
  spline S62 degree 2 poles (131.1513, -8.128) (131.9367, -8.128) (132.9964, -8.2984) (133.478, -8.6097) knots 0 0 0 1 2 2 2
  spline S63 degree 2 poles (133.478, -8.6097) (133.9597, -8.9209) (134.5154, -9.8916) (134.5154, -10.6104) knots 0 0 0 1 2 2 2
  spline S64 degree 2 poles (134.5154, -10.6104) (134.5154, -11.6107) (133.4928, -12.9668) (132.6185, -13.2928) knots 0 0 0 1 2 2 2
  line L135 (132.6185, -13.2928) -> (135.8715, -17.272)
  spline S65 degree 2 poles (133.2483, -10.7067) (133.2483, -10.3066) (132.9667, -9.6915) (132.6703, -9.4914) knots 0 0 0 1 2 2 2
  spline S66 degree 2 poles (132.6703, -9.4914) (132.411, -9.321) (131.7218, -9.1802) (131.218, -9.1802) knots 0 0 0 1 2 2 2
  line L136 (131.218, -9.1802) -> (130.0101, -9.1802)
  line L137 (130.0101, -9.1802) -> (130.0101, -12.6185)
  line L138 (130.0101, -12.6185) -> (131.0772, -12.6185)
  spline S67 degree 2 poles (131.0772, -12.6185) (131.6033, -12.6185) (132.4406, -12.4332) (132.7296, -12.1442) knots 0 0 0 1 2 2 2
  spline S68 degree 2 poles (132.7296, -12.1442) (132.9964, -11.8923) (133.2483, -11.1809) (133.2483, -10.7067) knots 0 0 0 1 2 2 2
  line L139 (135.6121, -17.272) -> (138.6947, -8.128)
  line L140 (138.6947, -8.128) -> (140.1915, -8.128)
  line L141 (140.1915, -8.128) -> (143.2741, -17.272)
  line L142 (143.2741, -17.272) -> (141.9922, -17.272)
  line L143 (141.9922, -17.272) -> (141.1622, -14.7155)
  line L144 (141.1622, -14.7155) -> (137.6721, -14.7155)
  line L145 (137.6721, -14.7155) -> (136.8422, -17.272)
  line L146 (136.8422, -17.272) -> (135.6121, -17.272)
  line L147 (140.8288, -13.6781) -> (139.4135, -9.3729)
  line L148 (139.4135, -9.3729) -> (138.0056, -13.6781)
  line L149 (138.0056, -13.6781) -> (140.8288, -13.6781)
  line L150 (150.6842, -17.272) -> (149.3207, -17.272)
  line L151 (149.3207, -17.272) -> (145.2748, -9.3877)
  line L152 (145.2748, -9.3877) -> (145.2748, -17.272)
  line L153 (145.2748, -17.272) -> (144.1411, -17.272)
  line L154 (144.1411, -17.272) -> (144.1411, -8.128)
  line L155 (144.1411, -8.128) -> (145.8676, -8.128)
  line L156 (145.8676, -8.128) -> (149.5504, -15.3676)
  line L157 (149.5504, -15.3676) -> (149.5504, -8.128)
  line L158 (149.5504, -8.128) -> (150.6842, -8.128)
  line L159 (150.6842, -8.128) -> (150.6842, -17.272)
  spline S69 degree 2 poles (155.0857, -17.435) (154.0928, -17.435) (152.6997, -17.0201) (152.0847, -16.7237) knots 0 0 0 1 2 2 2
  line L160 (152.0847, -16.7237) -> (152.0847, -15.1972)
  line L161 (152.0847, -15.1972) -> (152.1736, -15.1972)
  spline S70 degree 2 poles (152.1736, -15.1972) (152.7738, -15.7604) (154.2929, -16.3828) (154.9968, -16.3828) knots 0 0 0 1 2 2 2
  spline S71 degree 2 poles (154.9968, -16.3828) (156.0046, -16.3828) (157.0346, -15.5455) (157.0346, -14.8563) knots 0 0 0 1 2 2 2
  spline S72 degree 2 poles (157.0346, -14.8563) (157.0346, -14.308) (156.4936, -13.6263) (155.9082, -13.4558) knots 0 0 0 1 2 2 2
  spline S73 degree 2 poles (155.9082, -13.4558) (155.4859, -13.3373) (154.7819, -13.1742) (154.2558, -13.0409) knots 0 0 0 1 2 2 2
  spline S74 degree 2 poles (154.2558, -13.0409) (153.7816, -12.9149) (153.0331, -12.537) (152.7442, -12.2332) knots 0 0 0 1 2 2 2
  spline S75 degree 2 poles (152.7442, -12.2332) (152.4626, -11.9294) (152.1513, -11.1142) (152.1513, -10.5807) knots 0 0 0 1 2 2 2
  spline S76 degree 2 poles (152.1513, -10.5807) (152.1513, -9.4692) (153.8853, -7.965) (155.2265, -7.965) knots 0 0 0 1 2 2 2
  spline S77 degree 2 poles (155.2265, -7.965) (155.9972, -7.965) (157.3606, -8.2688) (157.946, -8.5578) knots 0 0 0 1 2 2 2
  line L162 (157.946, -8.5578) -> (157.946, -10.0102)
  line L163 (157.946, -10.0102) -> (157.8571, -10.0102)
  spline S78 degree 2 poles (157.8571, -10.0102) (157.4199, -9.61) (156.0564, -9.0172) (155.308, -9.0172) knots 0 0 0 1 2 2 2
  spline S79 degree 2 poles (155.308, -9.0172) (154.4633, -9.0172) (153.4185, -9.8101) (153.4185, -10.4548) knots 0 0 0 1 2 2 2
  spline S80 degree 2 poles (153.4185, -10.4548) (153.4185, -11.0327) (154.0335, -11.7219) (154.6115, -11.8775) knots 0 0 0 1 2 2 2
  spline S81 degree 2 poles (154.6115, -11.8775) (154.9968, -11.9812) (156.1157, -12.248) (156.4862, -12.3591) knots 0 0 0 1 2 2 2
  spline S82 degree 2 poles (156.4862, -12.3591) (157.4273, -12.6481) (158.3017, -13.8115) (158.3017, -14.6637) knots 0 0 0 1 2 2 2
  spline S83 degree 2 poles (158.3017, -14.6637) (158.3017, -15.2046) (157.8645, -16.242) (157.4718, -16.6051) knots 0 0 0 1 2 2 2
  spline S84 degree 2 poles (157.4718, -16.6051) (157.0346, -17.0052) (155.9231, -17.435) (155.0857, -17.435) knots 0 0 0 1 2 2 2
  line L164 (165.0078, -9.2099) -> (160.7544, -9.2099)
  line L165 (160.7544, -9.2099) -> (160.7544, -11.7886)
  line L166 (160.7544, -11.7886) -> (164.8299, -11.7886)
  line L167 (164.8299, -11.7886) -> (164.8299, -12.8704)
  line L168 (164.8299, -12.8704) -> (160.7544, -12.8704)
  line L169 (160.7544, -12.8704) -> (160.7544, -17.272)
  line L170 (160.7544, -17.272) -> (159.5392, -17.272)
  line L171 (159.5392, -17.272) -> (159.5392, -8.128)
  line L172 (159.5392, -8.128) -> (165.0078, -8.128)
  line L173 (165.0078, -8.128) -> (165.0078, -9.2099)
  spline S85 degree 2 poles (172.566, -9.1728) (173.0847, -9.7804) (173.6627, -11.5589) (173.6627, -12.7) knots 0 0 0 1 2 2 2
  spline S86 degree 2 poles (173.6627, -12.7) (173.6627, -13.8115) (173.0996, -15.6121) (172.566, -16.2198) knots 0 0 0 1 2 2 2
  spline S87 degree 2 poles (172.566, -16.2198) (172.0029, -16.857) (170.5134, -17.4647) (169.6168, -17.4647) knots 0 0 0 1 2 2 2
  spline S88 degree 2 poles (169.6168, -17.4647) (168.6906, -17.4647) (167.2086, -16.8348) (166.6676, -16.2198) knots 0 0 0 1 2 2 2
  spline S89 degree 2 poles (166.6676, -16.2198) (166.1415, -15.6121) (165.5784, -13.8263) (165.5784, -12.7) knots 0 0 0 1 2 2 2
  spline S90 degree 2 poles (165.5784, -12.7) (165.5784, -11.5514) (166.1489, -9.8027) (166.675, -9.1728) knots 0 0 0 1 2 2 2
  spline S91 degree 2 poles (166.675, -9.1728) (167.2086, -8.5652) (168.698, -7.9353) (169.6168, -7.9353) knots 0 0 0 1 2 2 2
  spline S92 degree 2 poles (169.6168, -7.9353) (170.5505, -7.9353) (172.0473, -8.5874) (172.566, -9.1728) knots 0 0 0 1 2 2 2
  spline S93 degree 2 poles (172.3956, -12.7) (172.3956, -11.796) (172.0029, -10.3955) (171.6472, -9.9361) knots 0 0 0 1 2 2 2
  spline S94 degree 2 poles (171.6472, -9.9361) (171.2841, -9.4618) (170.2615, -8.9876) (169.6242, -8.9876) knots 0 0 0 1 2 2 2
  spline S95 degree 2 poles (169.6242, -8.9876) (168.9647, -8.9876) (167.9718, -9.447) (167.5939, -9.9361) knots 0 0 0 1 2 2 2
  spline S96 degree 2 poles (167.5939, -9.9361) (167.2308, -10.4029) (166.8455, -11.8108) (166.8455, -12.7) knots 0 0 0 1 2 2 2
  spline S97 degree 2 poles (166.8455, -12.7) (166.8455, -14.5006) (168.3571, -16.4124) (169.6242, -16.4124) knots 0 0 0 1 2 2 2
  spline S98 degree 2 poles (169.6242, -16.4124) (170.8914, -16.4124) (172.3956, -14.5006) (172.3956, -12.7) knots 0 0 0 1 2 2 2
  line L174 (182.0731, -17.272) -> (180.4948, -17.272)
  line L175 (180.4948, -17.272) -> (177.6049, -13.6337)
  line L176 (177.6049, -13.6337) -> (176.2118, -13.6337)
  line L177 (176.2118, -13.6337) -> (176.2118, -17.272)
  line L178 (176.2118, -17.272) -> (174.9965, -17.272)
  line L179 (174.9965, -17.272) -> (174.9965, -8.128)
  line L180 (174.9965, -8.128) -> (177.3529, -8.128)
  spline S99 degree 2 poles (177.3529, -8.128) (178.1384, -8.128) (179.198, -8.2984) (179.6797, -8.6097) knots 0 0 0 1 2 2 2
  spline S100 degree 2 poles (179.6797, -8.6097) (180.1613, -8.9209) (180.7171, -9.8916) (180.7171, -10.6104) knots 0 0 0 1 2 2 2
  spline S101 degree 2 poles (180.7171, -10.6104) (180.7171, -11.6107) (179.6945, -12.9668) (178.8201, -13.2928) knots 0 0 0 1 2 2 2
  line L181 (178.8201, -13.2928) -> (182.0731, -17.272)
  spline S102 degree 2 poles (179.45, -10.7067) (179.45, -10.3066) (179.1684, -9.6915) (178.872, -9.4914) knots 0 0 0 1 2 2 2
  spline S103 degree 2 poles (178.872, -9.4914) (178.6126, -9.321) (177.9235, -9.1802) (177.4196, -9.1802) knots 0 0 0 1 2 2 2
  line L182 (177.4196, -9.1802) -> (176.2118, -9.1802)
  line L183 (176.2118, -9.1802) -> (176.2118, -12.6185)
  line L184 (176.2118, -12.6185) -> (177.2788, -12.6185)
  spline S104 degree 2 poles (177.2788, -12.6185) (177.8049, -12.6185) (178.6423, -12.4332) (178.9313, -12.1442) knots 0 0 0 1 2 2 2
  spline S105 degree 2 poles (178.9313, -12.1442) (179.198, -11.8923) (179.45, -11.1809) (179.45, -10.7067) knots 0 0 0 1 2 2 2
  line L185 (190.6391, -17.272) -> (189.4239, -17.272)
  line L186 (189.4239, -17.272) -> (189.4239, -9.3951)
  line L187 (189.4239, -9.3951) -> (187.0379, -14.7526)
  line L188 (187.0379, -14.7526) -> (186.2969, -14.7526)
  line L189 (186.2969, -14.7526) -> (183.933, -9.3951)
  line L190 (183.933, -9.3951) -> (183.933, -17.272)
  line L191 (183.933, -17.272) -> (182.7993, -17.272)
  line L192 (182.7993, -17.272) -> (182.7993, -8.128)
  line L193 (182.7993, -8.128) -> (184.4592, -8.128)
  line L194 (184.4592, -8.128) -> (186.7415, -13.2187)
  line L195 (186.7415, -13.2187) -> (188.9496, -8.128)
  line L196 (188.9496, -8.128) -> (190.6391, -8.128)
  line L197 (190.6391, -8.128) -> (190.6391, -17.272)
  dimension "d18" = 182.88
  dimension "d19" = 203.2
  dimension "d20" = 25.4
  dimension "d21" = 10.16
  dimension "d22" = 10.16
  dimension "d23" = 7.62
  constraints: 2 other
  measures "d18" distance of L0.start L0.end
  measures "d19" distance of L4.start L4.end
  measures "d20" distance of L4.start L5.end
  measures "d21" distance of L2.end L0.start
  measures "d22" distance between parallel lines of L5 L3
  measures "d23" distance between parallel lines of L6 L2
extrude "Extrusion4" cut sketch "Sketch4" against normal blind 5.08 contours L8 L9 L10 L11 L12 L13 S0 L14 L15 L16 L17 | L18 L19 S1 S2 S3 S4 S5 S6 L20 L21 S7 S8 S9 S10 S11 L22 L23 | L24 L25 L26 L27 | L28 L29 L30 L31 L32 L33 L34 L35 | S12 S13 S14 S15 S16 S17 S18 S19 | L36 L37 L38 L39 L40 L41 L42 L43 L44 L45 | L46 L47 L48 L49 L50 L51 L52 L53 L54 L55 L56 L57 | L58 L59 L60 L61 L62 L63 L64 L65 L66 L67 | S26 S27 S28 S29 S30 S31 S32 S33 | S40 S41 L68 L69 L70 S42 S43 S44 S45 L71 L72 L73 S46 S47 | L74 L75 L76 L77 L78 L79 L80 S48 S49 S50 L81 | L85 L86 L87 L88 L89 L90 L91 L92 L93 L94 L95 L96 | L97 L98 L99 L100 L101 L102 L103 L104 L105 L106 L107 L108 | L109 L110 L111 L112 L113 L114 L115 S55 S56 S57 L116 | L120 L121 L122 L123 L124 L125 L126 L127 | L128 L139 L135 | L135 L139 L140 L141 L142 L143 L144 L145 L146 | L128 L129 L130 L131 L132 L133 L134 S62 S63 S64 L135 L139 | L150 L151 L152 L153 L154 L155 L156 L157 L158 L159 | S69 L160 L161 S70 S71 S72 S73 S74 S75 S76 S77 L162 L163 S78 S79 S80 S81 S82 S83 S84 | L164 L165 L166 L167 L168 L169 L170 L171 L172 L173 | S85 S86 S87 S88 S89 S90 S91 S92 | L174 L175 L176 L177 L178 L179 L180 S99 S100 S101 L181 | L185 L186 L187 L188 L189 L190 L191 L192 L193 L194 L195 L196 L197